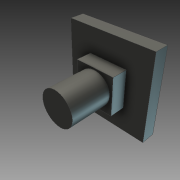
# Autodesk Inventor part: Camera - SONY CCD
Saved by Autodesk Inventor 2013 SP1 (Build 170176100, 176)
## iProperties
Created: 2013-03-14
Part Number: Camera - SONY CCD
Material: Generic
Document SubType Name: Modeling
Designer: fixer
Mass: 14.5 g
Surface Area: 51.4748 cm^2
Volume: 14.2199 cm^3
Density: 1.0197 g/cm^3
Author: fixer
Autodesk Inventor part; units mm, degrees
ref_plane "YZ Plane" through (0, 0, 0) normal (1, 0, 0) x (0, 1, 0)
ref_plane "XZ Plane" through (0, 0, 0) normal (0, 1, 0) x (-1, 0, 0)
ref_plane "XY Plane" through (0, 0, 0) normal (0, 0, 1) x (1, 0, 0)
sketch "Sketch1" plane through (0, 0, 0) normal (0, 0, 1) x (1, 0, 0)
  line L0 (19.05, -19.05) -> (-19.05, -19.05)
  line L1 (-19.05, -19.05) -> (-19.05, 19.05)
  line L2 (-19.05, 19.05) -> (19.05, 19.05)
  line L3 (19.05, 19.05) -> (19.05, -19.05)
  point P0 (0, 0)
  point P1 (-19.05, 0)
  point P2 (0, 19.05)
  dimension "d0" = 38.1
  dimension "d1" = 38.1
  constraints: 8 end point, 2 midpoint, 2 parallel, 1 horizontal, 1 horizontal alignment, 1 perpendicular, 1 vertical alignment
  measures "d0" distance of L0.end L1.end
  measures "d1" distance of L1.end L2.end
extrude "Extrusion1" add sketch "Sketch1" along normal blind 6.35
sketch "Sketch2" plane through (0, 0, 6.35) normal (0, 0, 1) x (1, 0, 0)
  line L0 (-19.05, -19.05) -> (-19.05, 19.05) projected
  line L1 (-19.05, 19.05) -> (19.05, 19.05) projected
  line L2 (8.636, -8.255) -> (-8.636, -8.255)
  line L3 (-8.636, -8.255) -> (-8.636, 8.255)
  line L4 (-8.636, 8.255) -> (8.636, 8.255)
  line L5 (8.636, 8.255) -> (8.636, -8.255)
  point P0 (0, 0)
  point P1 (0, 8.255)
  point P2 (0, 19.05)
  point P3 (-8.636, 0)
  point P4 (-19.05, 0)
  dimension "d4" = 17.272
  dimension "d5" = 16.51
  constraints: 8 end point, 4 midpoint, 2 parallel, 1 horizontal, 1 horizontal alignment, 1 perpendicular, 1 vertical alignment
  measures "d4" distance of L3.end L4.end
  measures "d5" distance of L4.end L2.start
extrude "Extrusion2" add sketch "Sketch2" along normal blind 6.858
sketch "Sketch3" plane through (0, 0, 13.208) normal (0, 0, 1) x (1, 0, 0)
  circle A0 centre (0, 0) radius 7.493
  point P0 (0, 0)
  dimension "d8" = 14.986
  constraints: 1 centre point, 1 coincident
  measures "d8" diameter of A0
extrude "Extrusion3" add sketch "Sketch3" along normal blind 17.272
body "Solid1"
